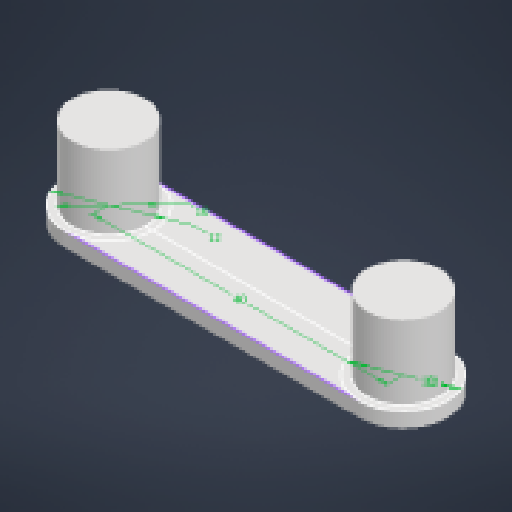
# Autodesk Inventor part: Test
Saved by Autodesk Inventor 2026.2 (Build 302298000, 298)
## iProperties
Created: 2025-12-17
Part Number: Test
Material: Generic
Document SubType Name: Modeling
Designer: Cobble
Density: 1 g/cm^3
Appearance: Default
Author: Cobble
Autodesk Inventor part; units mm, degrees
ref_plane "YZ Plane" through (0, 0, 0) normal (1, 0, 0) x (0, 1, 0)
ref_plane "XZ Plane" through (0, 0, 0) normal (0, 1, 0) x (-1, 0, 0)
ref_plane "XY Plane" through (0, 0, 0) normal (0, 0, 1) x (1, 0, 0)
sketch "Sketch1" plane through (0, 0, 0) normal (0, 0, 1) x (1, 0, 0)
  circle A0 centre (0, 0) radius 5
  circle A1 centre (0, 0) radius 6
  line L0 (0, 0) -> (-40, 0)
  circle A2 centre (-40, 0) radius 5
  circle A3 centre (-40, 0) radius 6
  line L1 (-40, 6) -> (0, 6)
  line L2 (0, -6) -> (-40, -6)
  dimension "d0" = 10
  dimension "d1" = 12
  dimension "d2" = 40
  dimension "d3" = 10
  dimension "d4" = 12
  constraints: 6 end point, 4 centre point, 4 coincident, 4 point on circle, 2 tangent, 1 horizontal
  measures "d0" diameter of A0
  measures "d1" diameter of A1
  measures "d2" distance of L0.start L0.end
  measures "d3" diameter of A2
  measures "d4" diameter of A3
extrude "Extrusion1" add sketch "Sketch1" along normal blind 10 contours A0 | A2
extrude "Extrusion2" add sketch "Sketch1" against normal blind 2 contours A0 | A1 | A1 L2 A3 L0 | L0 A3 L1 A1 | A2 | A3
body "Solid1"
